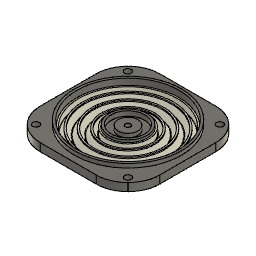
Passive_radiator_ND65-PR_compatible (Autodesk Fusion 360 design; units mm, degrees)
Autodesk Fusion 360 part; units mm, degrees
note: some values were not read from the file. Set by a fixed rule: which sketch regions a step uses.
sketch "Sketch1" plane through (0, 0, 0) normal (1, 0, 0) x (0, 1, 0)
  line L0 (0, 0) -> (-1.2, 0)
  line L1 (-1.2, 0) -> (-1.2, 3)
  line L2 (-1.2, 3) -> (0, 3)
  line L3 (0, 3) -> (0, 0)
  line L4 (0, 0) -> (4, 0)
  line L5 (4, 0) -> (4, 0.8)
  line L6 (4, 0.8) -> (0, 0.8)
  line L7 (0, 0.8) -> (0, 0)
  dimension "d1" = 1.2
  dimension "d2" = 3
  dimension "d3" = 4
  dimension "d4" = 0.8
  constraint horizontal L0
  constraint vertical L1
  constraint horizontal L2
  constraint vertical L3
  constraint coincident L0.start L3.end
  constraint horizontal L4
  constraint vertical L5
  constraint horizontal L6
  constraint vertical L7
  measures "d1" distance of L1.end L2.end
  measures "d2" distance of L0.start L2.end
  measures "d3" distance of L0.start L4.end
  measures "d4" distance of L0.start L6.end
sketch "Sketch1 (2)" plane through (0, 0, 0) normal (1, 0, 0) x (0, 1, 0) in component "surround"
  line L0 (3, 0.6) -> (0, 0.6)
  line L1 (0, 0) -> (3, 0)
  line L2 (-0.8, 0) -> (-0.8, 3.5)
  line L3 (0, 3.5) -> (0, 0)
  line L4 (0, 0) -> (-0.8, 0)
  line L5 (0, 0.6) -> (0, 0)
  line L6 (3, 0) -> (3, 0.6)
  line L7 (-0.8, 3.5) -> (0, 3.5)
  line L8 (-0.8, 0.6) -> (-0.8, 0)
  line L9 (-1.2, 0) -> (-3.2, 2.3835)
  line L10 (-1.2, 0) -> (1.0702, 0) construction
  line L11 (-2.8, 2.3835) -> (-0.8, 0)
  line L12 (-3.2, 2.3835) -> (-5.2, 0)
  line L13 (-5.6, 0) -> (-3.6, 2.3835)
  line L14 (-5.2, 0) -> (-5.6, 0)
  line L15 (-1.2, 0) -> (-0.8, 0)
  line L16 (-2.8, 2.3835) -> (-3.6, 2.3835) construction
  line L17 (-3.6, 2.3835) -> (-3.6, 2.9835)
  line L18 (-3.6, 2.9835) -> (-2.8, 2.9835)
  line L19 (-2.8, 2.9835) -> (-2.8, 2.3835)
  line L20 (-5.6, 0) -> (-5.6, 0.4) construction
  line L21 (-5.6, 0.4) -> (-5.2644, 0.4) construction
  line L22 (-1.1356, 0.4) -> (-0.8, 0.4) construction
  line L23 (-10.4, 0) -> (-8.4, 2.3835)
  line L24 (-8, 2.3835) -> (-10, 0)
  line L25 (-10.4, 0.4) -> (-10.0644, 0.4) construction
  line L26 (-10, 0) -> (-10.4, 0)
  line L27 (-6, 0) -> (-5.6, 0)
  line L28 (-6, 0) -> (-8, 2.3835)
  line L29 (-7.6, 2.3835) -> (-5.6, 0)
  line L30 (-5.9356, 0.4) -> (-5.6, 0.4) construction
  line L31 (-7.6, 2.9835) -> (-7.6, 2.3835)
  line L32 (-8.4, 2.9835) -> (-7.6, 2.9835)
  line L33 (-8.4, 2.3835) -> (-8.4, 2.9835)
  line L34 (-8, 0.3835) -> (-8, 2.3835) construction
  line L35 (-15.2, 0) -> (-15.2, 3.5)
  line L36 (-16, 3.5) -> (-16, 0)
  line L37 (-19, 0.6) -> (-16, 0.6)
  line L38 (-16, 0) -> (-19, 0)
  line L39 (-16, 0) -> (-15.2, 0)
  line L40 (-19, 0) -> (-19, 0.6)
  line L41 (-15.2, 3.5) -> (-16, 3.5)
  line L42 (-25.8, 0.0014) -> (-25.8, 10.0014)
  line L43 (-15.2, 0) -> (-13.2, 2.3835)
  line L44 (-12.8, 2.3835) -> (-14.8, 0)
  line L45 (-15.2, 0.4) -> (-14.8644, 0.4)
  line L46 (-14.8, 0) -> (-15.2, 0)
  line L47 (-10.8, 0) -> (-10.4, 0)
  line L48 (-10.8, 0) -> (-12.8, 2.3835)
  line L49 (-12.4, 2.3835) -> (-10.4, 0)
  line L50 (-10.7356, 0.4) -> (-10.4, 0.4) construction
  line L51 (-12.4, 2.9835) -> (-12.4, 2.3835)
  line L52 (-13.2, 2.9835) -> (-12.4, 2.9835)
  line L53 (-13.2, 2.3835) -> (-13.2, 2.9835)
  line L54 (-1.2, 0) -> (3, 0)
  line L55 (3, 0) -> (3, -0.6)
  line L56 (3, -0.6) -> (-1.2, -0.6)
  line L57 (-1.2, -0.6) -> (-1.2, 0)
  line L58 (-5.2, 0) -> (-6, 0)
  line L59 (-6, 0) -> (-6, -0.6)
  line L60 (-6, -0.6) -> (-5.2, -0.6)
  line L61 (-5.2, -0.6) -> (-5.2, 0)
  line L62 (-10.8, 0) -> (-10, 0)
  line L63 (-10, 0) -> (-10, -0.6)
  line L64 (-10, -0.6) -> (-10.8, -0.6)
  line L65 (-10.8, -0.6) -> (-10.8, 0)
  line L66 (-14.8, 0) -> (-19, 0)
  line L67 (-19, 0) -> (-19, -0.6)
  line L68 (-19, -0.6) -> (-14.8, -0.6)
  line L69 (-14.8, -0.6) -> (-14.8, 0)
  dimension "d5" = 0.8
  dimension "d6" = 3.5
  dimension "d7" = 3
  dimension "d8" = 0.6
  dimension "d9" = 0.4
  dimension "d10" = 0.6
  dimension "d11" = 130
  dimension "d12" = 2
  dimension "d13" = 0.4
  dimension "d14" = 50
  dimension "d15" = 0.4
  dimension "d16" = 0.6
  dimension "d17" = 0.4
  dimension "d18" = 0.4
  dimension "d21" = -4.8
  dimension "d22" = 0
  dimension "d24" = 10
  dimension "d25" = 25.8
  dimension "d63" = 2
  dimension "d64" = 0.6
  dimension "d65" = 0.6
  dimension "d66" = 0.6
  dimension "d67" = 0.6
  constraint horizontal L4
  constraint vertical L2
  constraint horizontal L7
  constraint vertical L3
  constraint coincident L1.start L3.end
  constraint horizontal L1
  constraint vertical L6
  constraint horizontal L0
  constraint vertical L5
  constraint vertical L8
  constraint horizontal L10
  constraint coincident L10 L2.start
  constraint parallel L9 L11
  constraint horizontal L9.end L11.start
  constraint horizontal L9.end L13.end
  constraint horizontal L12.end L13.start
  constraint equal L12 L13
  constraint horizontal L1.start L9.start
  constraint coincident L1.start L14
  constraint horizontal L16
  constraint vertical L17
  constraint horizontal L18
  constraint vertical L19
  constraint coincident L13.end L17
  constraint vertical L20
  constraint coincident L13 L21.end
  constraint perpendicular L20 L21
  constraint coincident L11 L22.start
  constraint horizontal L22
  constraint vertical L2.start L22.end
  constraint symmetric L0.end L34 L37.end
  constraint symmetric L1.end L34 L38.end
  constraint symmetric L0.start L34 L37.start
  constraint symmetric L1.start L34 L36.end
  constraint symmetric L3.start L34 L36.start
  constraint symmetric L2.end L34 L35.end
  constraint symmetric L2.start L34 L35.start
  constraint perpendicular L37 L42
  constraint horizontal L23.start L38.end
  constraint vertical L34
  constraint horizontal L54
  constraint vertical L55
  constraint horizontal L56
  constraint vertical L57
  constraint horizontal L58
  constraint vertical L59
  constraint horizontal L60
  constraint vertical L61
  constraint horizontal L62
  constraint vertical L63
  constraint horizontal L64
  constraint vertical L65
  constraint horizontal L66
  constraint vertical L67
  constraint horizontal L68
  constraint vertical L69
  measures "d5" distance of L3.start L2.end
  measures "d6" distance of L1.start L3.start
  measures "d7" distance of L1.end L1.start
  measures "d8" distance of L0.end L1.start
  measures "d9" distance of L2.start L9.start
  measures "d10" distance of L2.start L8.start
  measures "d11" angle of L9 L10
  measures "d12" horizontal distance of L9.start L9.end
  measures "d13" distance of L9.end L11.start
  measures "d14" angle of L4 L12
  measures "d15" distance of L9.end L13.end
  measures "d16" distance of L11.start L18.end
  measures "d17" distance of L13.start L20.end
  measures "d18" vertical distance of L2.start L22.end
  measures "d24" distance of L42.start L42.end
  measures "d25" distance of L1.start L42
  measures "d63" distance of L24.start L34.start
  measures "d64" distance of L9.start L56.end
  measures "d65" distance of L12.end L60.end
  measures "d66" distance of L47.start L64.end
  measures "d67" distance of L44.end L68.end
revolve "Revolve1" add sketch "Sketch1 (2)" angle 360 about axis through (0, -25.8, 0.0014) along (0, 0, 1) contours L2 L3 L4 L5 L7 L8 L54 | L1 L4 L15 L54 L55 L56 L57 | L9 L11 L12 L13 L14 L15 L17 L18 L19 L54 L58 | L14 L27 L58 L59 L60 L61 | L23 L24 L26 L27 L28 L29 L31 L32 L33 L58 L62 | L26 L47 L62 L63 L64 L65 | L43 L44 L46 L47 L48 L49 L51 L52 L53 L62 L66 | L38 L39 L46 L66 L67 L68 L69 | L35 L36 L39 L41 L66 | L35 L43 L45 makes body 1 in component "surround"
chamfer "Chamfer1" distance 0.5 angle 45 2 edges at (-6.3398, -23.341, -0.6) (-26.851, -15.3855, -0.6) on bodies 1 in component "surround"
sketch "Sketch1 (3)" plane through (0, 0, 0) normal (1, 0, 0) x (0, 1, 0) in component "Hard bits"
  line L0 (-25.8, 0.0014) -> (-25.8, 10.0014)
  line L1 (-19, 0.6) -> (-16, 0.6)
  line L2 (-16, 3.5) -> (-16, 0)
  line L3 (0, 3.5) -> (0, 0)
  line L4 (3, 0.6) -> (0, 0.6)
  line L5 (-16.15, 3.5) -> (-16.15, 0)
  line L6 (0.15, 3.5) -> (0.15, 0)
  line L7 (0.15, 0.6) -> (1.35, 0.6)
  line L8 (1.35, 0.6) -> (1.35, 6.6)
  line L9 (1.35, 6.6) -> (0.15, 6.6)
  line L10 (0.15, 6.6) -> (0.15, 0.6)
  line L11 (1.35, 0.6) -> (10.35, 0.6)
  line L12 (10.35, 0.6) -> (10.35, 4.6)
  line L13 (10.35, 4.6) -> (1.35, 4.6)
  line L14 (1.35, 4.6) -> (1.35, 0.6)
  line L15 (-16.15, 0.6) -> (-25.8, 0.6)
  line L16 (-25.8, 0.6) -> (-25.8, 4.6)
  line L17 (-25.8, 4.6) -> (-16.15, 4.6)
  line L18 (-16.15, 4.6) -> (-16.15, 0.6)
  line L19 (-25.8, 4.6) -> (-17.35, 4.6)
  line L20 (-17.35, 4.6) -> (-17.35, 2.2)
  line L21 (-17.35, 2.2) -> (-25.8, 2.2)
  line L22 (-25.8, 2.2) -> (-25.8, 4.6)
  dimension "d28" = 0.15
  dimension "d29" = -0.15
  dimension "d30" = 1.2
  dimension "d31" = 6
  dimension "d32" = 9
  dimension "d33" = 4
  dimension "d34" = 4
  dimension "d35" = 1.2
  dimension "d36" = 1.6
  constraint horizontal L7
  constraint vertical L8
  constraint horizontal L9
  constraint vertical L10
  constraint coincident L4 L7.start
  constraint coincident L6 L7.start
  constraint horizontal L11
  constraint vertical L12
  constraint horizontal L13
  constraint vertical L14
  constraint horizontal L15
  constraint vertical L16
  constraint horizontal L17
  constraint vertical L18
  constraint collinear L0 L16
  constraint horizontal L19
  constraint vertical L20
  constraint horizontal L21
  constraint vertical L22
  constraint collinear L5 L18
  constraint collinear L1 L15
  measures "d30" distance of L7.start L7.end
  measures "d31" distance of L7.start L9.end
  measures "d32" distance of L7.end L11.end
  measures "d33" distance of L7.end L13.end
  measures "d34" distance of L15.start L17.end
  measures "d35" distance of L18 L20
  measures "d36" distance of L15 L21
revolve "Revolve1'" add sketch "Sketch1 (3)" angle 360 about axis through (0, -25.8, 0.6) along (0, 0, 1) separate body contours L0 L1 L5 L15 L16 L17 L18 L20 L21 makes body 2 in component "Hard bits"
revolve "Revolve2" add sketch "Sketch1 (3)" angle 360 about axis through (0, -25.8, 0.6) along (0, 0, 1) separate body contours L4 L8 L11 L12 L13 L14 | L4 L6 L7 L8 L9 L10 L14 makes body 3 in component "Hard bits"
sketch "Sketch2" plane through (0, 0, 4.6) normal (0, 0, 1) x (-1, 0, 0) in component "Hard bits"
  circle A0 centre (0, 25.8) radius 27.15
  circle A1 centre (0, 25.8) radius 36.15
  circle A2 centre (0, 25.8) radius 33 construction
  circle A3 centre (-23.3345, 2.4655) radius 1.7
  circle A4 centre (23.3345, 2.4655) radius 1.7
  circle A5 centre (23.3345, 49.1345) radius 1.7
  circle A6 centre (-23.3345, 49.1345) radius 1.7
  line L0 (-23.3345, 2.4655) -> (0, 25.8)
  line L1 (0, 25.8) -> (0, 17.35)
  line L2 (-30.3, 56.1) -> (30.3, 56.1)
  line L3 (30.3, 56.1) -> (30.3, -4.5)
  line L4 (30.3, -4.5) -> (-30.3, -4.5)
  line L5 (-30.3, -4.5) -> (-30.3, 56.1)
  line L6 (-30.3, 56.1) -> (30.3, -4.5) construction
  line L7 (30.3, 56.1) -> (-30.3, -4.5) construction
  point P0 (0, 25.8)
  dimension "d39" = 66
  dimension "d40" = 3.4
  dimension "d42" = 360
  dimension "d58" = 45
  dimension "d59" = 60.6
  dimension "d60" = 60.6
  constraint concentric A0 A2
  constraint coincident A2 A3.centre
  constraint coincident A3.centre L0.start
  constraint coincident P0 A0.centre
  constraint horizontal L2
  constraint perpendicular L2 L3
  constraint parallel L2 L4
  constraint parallel L3 L5
  constraint coincident L6 P0
  constraint coincident L7 P0
  measures "d39" diameter of A2
  measures "d40" diameter of A3
  measures "d58" angle of L0 L1
  measures "d59" distance of L2.end L3.end
  measures "d60" distance of L2.start L2.end
extrude "Extrude1" cut sketch "Sketch2" against normal up to surface (4 mm away) contours A3 | A4 | A5 | A6 bodies 3 in component "Hard bits"
sketch "Sketch3" plane through (0, 0, 2.2) normal (0, 0, 1) x (-1, 0, 0) in component "Hard bits"
  circle A0 centre (0, 25.8) radius 8.45
  circle A1 centre (0, 25.8) radius 5
  circle A2 centre (0, 25.8) radius 1.35
  dimension "d45" = 10
  dimension "d46" = 2.7
  constraint concentric A0 A1
  constraint concentric A1 A2
  measures "d45" diameter of A1
  measures "d46" diameter of A2
extrude "Extrude2" add sketch "Sketch3" along normal blind 2 contours A1 bodies 2 in component "Hard bits"
extrude "Extrude3" cut 1 faces at (-0.3499, -25.6266, 2.2) along direction (0, 0, -1) up to surface (1.2 mm away) on bodies 2 bodies 2 in component "Hard bits"
sketch "Sketch4" plane through (0, 0, 0) normal (0, 1, 0) x (1, 0, 0) in component "Hard bits"
  circle A0 centre (0, -2.6) radius 2.5
  line L0 (0, -0.6) -> (0, -4.6)
  dimension "d51" = 5
  constraint midpoint A0.centre L0
  measures "d51" diameter of A0
extrude "Extrude4" [suppressed] in component "Hard bits"
pattern_circular "C-Pattern1" [suppressed] in component "Hard bits"
extrude "Extrude5" cut sketch "Sketch2" along normal mid plane 21.2878 contours A0 | A1 L2 L3 L4 L5 keep common part bodies 3 in component "Hard bits"
extrude "Extrude6" cut 1 faces at (-0.3499, -25.6266, 1) along direction (0, 0, -1) up to surface (0.4 mm away) on bodies 2 bodies 2 in component "Hard bits"
fillet "Fillet1" radius 16 8 edges at (19.7163, -56.1, 2.6) (30.3, -45.5163, 2.6) (-19.7163, -56.1, 2.6) (-30.3, -45.5163, 2.6) (-30.3, -6.0837, 2.6) (-19.7163, 4.5, 2.6) (19.7163, 4.5, 2.6) (30.3, -6.0837, 2.6) on bodies 3 in component "Hard bits"
component "surround" placed x (1, 0, 0) y (0, 1, 0) z (0, 0, 1) at (0, 0, 0)
component "Hard bits" placed x (1, 0, 0) y (0, 1, 0) z (0, 0, 1) at (0, 0, 0)
named bodies: "Surround", "inner", "outer"
